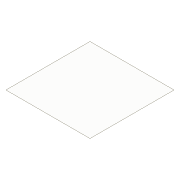
# Autodesk Inventor part: Diffusionsfolie 460x460
Saved by Autodesk Inventor 2021.3 (Build 253353000, 353)
## iProperties
Part Number: Diffusionsfolie 460x460
Material: PA 6.6
Document SubType Name: Modeling
Designer: SRORF
Mass: 24.1224 g
Surface Area: 4233.84 cm^2
Volume: 21.16 cm^3
Density: 1.14 g/cm^3
Appearance: Lexan (rauch)
Author: SRORF
ROT_Density: 1.0
PDB_Ident_Ver: =<PDB_Ident> <PDB_Version>
ROT_Weight: 0.024 kg
ROT_Weight_Num: 0.02412240000000001
Autodesk Inventor part; units mm, degrees
ref_plane "YZ Plane" through (0, 0, 0) normal (1, 0, 0) x (0, 1, 0)
ref_plane "XZ Plane" through (0, 0, 0) normal (0, 1, 0) x (-1, 0, 0)
ref_plane "XY Plane" through (0, 0, 0) normal (0, 0, 1) x (1, 0, 0)
sketch "Skizze2" plane through (0, 0, 0) normal (0, 0, 1) x (1, 0, 0)
  line L0 (-230, 230) -> (230, 230)
  line L1 (230, 230) -> (230, -230)
  line L2 (230, -230) -> (-230, -230)
  line L3 (-230, -230) -> (-230, 230)
  point P0 (0, 0)
  point P1 (0, 230)
  point P2 (-230, 0)
  dimension "d0" = 460
  dimension "d1" = 460
  constraints: 8 end point, 2 midpoint, 2 parallel, 1 horizontal, 1 horizontal alignment, 1 perpendicular, 1 vertical alignment
  measures "d0" distance of L2.end L0.start
  measures "d1" distance of L0.start L0.end
extrude "Extrusion1" add sketch "Skizze2" along normal blind 0.1
